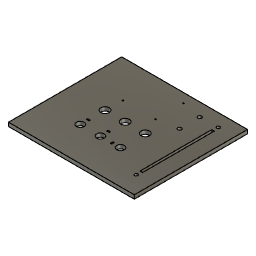
Case - Boden v14 (Autodesk Fusion 360 archive; units mm, degrees)
design "Case - Front"
Autodesk Fusion 360 part; units mm, degrees
sketch "sketch 319" plane through (0, 0, 0) normal (0, 0, 1) x (1, 0, 0)
  line L0 (0, 90) -> (100.0026, 90)
  line L1 (100.0026, 90) -> (100.0026, -0.0023)
  line L2 (100.0026, -0.0023) -> (0, -0.0023)
  line L3 (0, -0.0023) -> (0, 90)
  line L4 (24.0006, 83.9998) -> (75.0019, 83.9998)
  line L5 (75.0019, 83.9998) -> (75.0019, 58.9992)
  line L6 (75.0019, 58.9992) -> (24.0006, 58.9992)
  line L7 (24.0006, 58.9992) -> (24.0006, 83.9998)
  line L8 (78.8465, 82.9579) -> (94.847, 82.9579)
  line L9 (94.847, 82.9579) -> (94.847, 10.956)
  line L10 (94.847, 10.956) -> (78.8465, 10.956)
  line L11 (78.8465, 10.956) -> (78.8465, 82.9579)
  circle A0 centre (86.9203, 14.6115) radius 1.25
  circle A1 centre (86.9203, 79.8121) radius 1.25
  line L12 (85.9203, 75.7085) -> (87.9203, 75.7085)
  line L13 (87.9203, 75.7085) -> (87.9203, 18.707)
  line L14 (87.9203, 18.707) -> (85.9203, 18.707)
  line L15 (85.9203, 18.707) -> (85.9203, 75.7085)
  circle A2 centre (30.0768, 46.6723) radius 3.3501
  circle A3 centre (46.0772, 46.6723) radius 3.3501
  circle A4 centre (62.0776, 46.6723) radius 3.3501
  circle A5 centre (30.0268, 27.0218) radius 3.0001
  circle A6 centre (46.0272, 27.0218) radius 3.0001
  circle A7 centre (62.0276, 27.0218) radius 3.0001
  line L16 (29.0007, 33.9986) -> (31.0008, 33.9986)
  line L17 (31.0008, 33.9986) -> (31.0008, 32.9985)
  line L18 (31.0008, 32.9985) -> (29.0007, 32.9985)
  line L19 (29.0007, 32.9985) -> (29.0007, 33.9986)
  line L20 (45.0012, 33.9986) -> (47.0012, 33.9986)
  line L21 (47.0012, 33.9986) -> (47.0012, 32.9985)
  line L22 (47.0012, 32.9985) -> (45.0012, 32.9985)
  line L23 (45.0012, 32.9985) -> (45.0012, 33.9986)
  line L24 (56.0014, 27.9984) -> (56.0014, 25.9983)
  line L25 (56.0014, 25.9983) -> (55.0014, 25.9983)
  line L26 (55.0014, 25.9983) -> (55.0014, 27.9984)
  line L27 (55.0014, 27.9984) -> (56.0014, 27.9984)
  circle A8 centre (72.5019, 79.4997) radius 1.5
  circle A9 centre (72.5019, 63.4993) radius 1.5
  circle A10 centre (56.5015, 82.4998) radius 0.5
  circle A11 centre (56.5015, 60.4992) radius 0.5
  circle A12 centre (30.5008, 60.5171) radius 0.5
extrude "Extrusion1" add sketch "sketch 319" along normal blind 3 contours L0 L1 L2 L3 | L4 L5 L6 L7 | L8 L9 L10 L11
